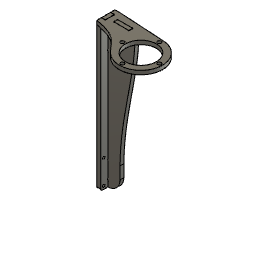
HoseSupport v3 (Autodesk Fusion 360 design; units mm, degrees)
Autodesk Fusion 360 part; units mm, degrees
sketch "Sketch1" plane through (0, 0, 0) normal (1, 0, 0) x (0, 0, -1)
  line L0 (0, 0) -> (10, 0) construction
  line L1 (10, 0) -> (50, 0) construction
  line L2 (10, 0) -> (10, 80) construction
  line L3 (50, 0) -> (50, 80) construction
  line L4 (0, 0) -> (0, -10) construction
  line L5 (0, 0) -> (0, 90) construction
  line L6 (0, 0) -> (60, 0) construction
  line L7 (60, 0) -> (60, 457.2) construction
  line L8 (0, -10) -> (60, -10)
  line L9 (60, -10) -> (60, 457.2)
  line L10 (60, 457.2) -> (0, 457.2)
  line L11 (0, 457.2) -> (0, -10)
  circle A0 centre (10, 80) radius 4
  circle A1 centre (50, 80) radius 4
  circle A2 centre (10, 0) radius 4
  circle A3 centre (50, 0) radius 4
  line L12 (30, -10) -> (30, 40) construction
  line L13 (36.35, 10) -> (23.65, 10)
  line L14 (23.65, 10) -> (23.65, 70)
  line L15 (23.65, 70) -> (36.35, 70)
  line L16 (36.35, 70) -> (36.35, 10)
  line L17 (36.35, 10) -> (23.65, 70) construction
  line L18 (23.65, 10) -> (36.35, 70) construction
  line L19 (30, 457.2) -> (30, 407.2) construction
  line L20 (36.35, 377.2) -> (23.65, 377.2)
  line L21 (23.65, 377.2) -> (23.65, 437.2)
  line L22 (23.65, 437.2) -> (36.35, 437.2)
  line L23 (36.35, 437.2) -> (36.35, 377.2)
  line L24 (36.35, 377.2) -> (23.65, 437.2) construction
  line L25 (23.65, 377.2) -> (36.35, 437.2) construction
  line L26 (0, 457.2) -> (15, 457.2) construction
  line L27 (60, 457.2) -> (45, 457.2) construction
  line L28 (45, 457.2) -> (45, 469.9) construction
  line L29 (15, 457.2) -> (45, 457.2)
  line L30 (45, 457.2) -> (45, 469.9)
  line L31 (45, 469.9) -> (15, 469.9)
  line L32 (15, 469.9) -> (15, 457.2)
  point P0 (30, 40)
  point P1 (30, 407.2)
  dimension "d1" = 10
  dimension "d2" = 40
  dimension "d3" = 80
  dimension "d4" = 80
  dimension "d5" = 10
  dimension "d6" = 90
  dimension "d8" = 60
  dimension "d9" = 457.2
  dimension "d10" = 8
  dimension "d11" = 8
  dimension "d12" = 8
  dimension "d13" = 8
  dimension "d14" = 50
  dimension "d15" = 12.7
  dimension "d16" = 60
  dimension "d17" = 50
  dimension "d18" = 12.7
  dimension "d19" = 60
  dimension "d20" = 15
  dimension "d21" = 15
  dimension "d22" = 12.7
  constraint coincident L0.start L4.start
  constraint horizontal L0
  constraint parallel L0 L1
  constraint perpendicular L1 L2
  constraint perpendicular L1 L3
  constraint perpendicular L0 L4
  constraint vertical L5
  constraint perpendicular L3 L6
  constraint perpendicular L6 L7
  constraint horizontal L8
  constraint vertical L9
  constraint horizontal L10
  constraint vertical L11
  constraint coincident L2.end A0.centre
  constraint coincident L3.end A1.centre
  constraint coincident L0.end L1.start
  constraint coincident L1.end L3.start
  constraint midpoint L8 L12.start
  constraint perpendicular L8 L12
  constraint horizontal L13
  constraint perpendicular L13 L14
  constraint parallel L13 L15
  constraint parallel L14 L16
  constraint coincident L17 P0
  constraint coincident L18 P0
  constraint coincident P0 L12.end
  constraint midpoint L10 L19.start
  constraint perpendicular L10 L19
  constraint horizontal L20
  constraint perpendicular L20 L21
  constraint parallel L20 L22
  constraint parallel L21 L23
  constraint coincident L24 P1
  constraint coincident L25 P1
  constraint coincident P1 L19.end
  constraint perpendicular L9 L26
  constraint perpendicular L9 L27
  constraint perpendicular L27 L28
  constraint horizontal L29
  constraint vertical L30
  constraint horizontal L31
  constraint vertical L32
  measures "d1" distance of L0.start L0.end
  measures "d2" distance of L0.end L1.end
  measures "d3" distance of L0.end L2.end
  measures "d4" distance of L1.end L3.end
  measures "d5" distance of L0.start L4.end
  measures "d6" distance of L0.start L5.end
  measures "d8" distance of L0.start L6.end
  measures "d9" distance of L6.end L7.end
  measures "d10" diameter of A0
  measures "d11" diameter of A1
  measures "d12" diameter of A2
  measures "d13" diameter of A3
  measures "d14" distance of L12.start P0
  measures "d15" distance of L14.end L15.end
  measures "d16" distance of L13.end L14.end
  measures "d17" distance of L19.start P1
  measures "d18" distance of L21.end L22.end
  measures "d19" distance of L20.end L21.end
  measures "d20" distance of L10.end L26.end
  measures "d21" distance of L7.end L27.end
  measures "d22" distance of L27.end L28.end
extrude "Extrude1" add sketch "Sketch1" along normal blind 12.7 makes body 1 in component "Component"
fillet "Fillet1" radius 6 2 edges at (6.35, -10, 0) (6.35, -10, -60) on bodies 1 in component "Component"
sketch "Sketch2" plane through (12.7, 0, 0) normal (1, 0, 0) x (0, 0, -1)
  arc A0 (54, -10) -> (60, -4) centre (54, -4) ccw
  line L0 (60, -4) -> (60, 457.2)
  line L1 (60, 457.2) -> (45, 457.2)
  line L2 (45, 457.2) -> (45, 469.9)
  line L3 (45, 469.9) -> (15, 469.9)
  line L4 (15, 469.9) -> (15, 457.2)
  line L5 (15, 457.2) -> (0, 457.2)
  line L6 (0, 457.2) -> (0, -4)
  arc A1 (0, -4) -> (6, -10) centre (6, -4) ccw
  line L7 (6, -10) -> (54, -10)
  circle A2 centre (50, 0) radius 4
  line L8 (23.65, 437.2) -> (36.35, 437.2)
  line L9 (36.35, 437.2) -> (36.35, 377.2)
  line L10 (36.35, 377.2) -> (23.65, 377.2)
  line L11 (23.65, 377.2) -> (23.65, 437.2)
  circle A3 centre (50, 80) radius 4
  circle A4 centre (10, 80) radius 4
  circle A5 centre (10, 0) radius 4
  line L12 (23.65, 70) -> (36.35, 70)
  line L13 (36.35, 70) -> (36.35, 10)
  line L14 (36.35, 10) -> (23.65, 10)
  line L15 (23.65, 10) -> (23.65, 70)
  line L16 (30, -10) -> (30, 223.6) construction
  line L17 (36.35, -10) -> (23.65, -10)
  line L18 (23.65, -10) -> (23.65, 457.2)
  line L19 (23.65, 457.2) -> (36.35, 457.2)
  line L20 (36.35, 457.2) -> (36.35, -10)
  line L21 (36.35, -10) -> (23.65, 457.2) construction
  line L22 (23.65, -10) -> (36.35, 457.2) construction
  point P0 (30, 223.6)
  dimension "d27" = 233.6
  dimension "d28" = 12.7
  constraint midpoint L7 L16.start
  constraint perpendicular L3 L16
  constraint horizontal L17
  constraint perpendicular L17 L18
  constraint parallel L17 L19
  constraint parallel L18 L20
  constraint coincident L21 P0
  constraint coincident L22 P0
  constraint coincident P0 L16.end
  measures "d27" distance of L16.start P0
  measures "d28" distance of L18.end L19.end
extrude "Extrude1'" add sketch "Sketch2" along normal blind 40 separate body contours L7 L14 L17 L18 L20 | L12 L13 L14 L15 L18 L20 | L10 L12 L18 L20 | L8 L9 L10 L11 L18 L20 | L8 L18 L19 L20 makes body 2 in component "Component'"
extrude "Extrude2" add sketch "Sketch2" against normal blind 12.7 contours L12 L13 L14 L15 L18 L20 | L8 L9 L10 L11 L18 L20 bodies 2 in component "Component'"
sketch "Sketch3" plane through (0, 0, -23.65) normal (0, 0, 1) x (1, 0, 0)
  line L0 (12.7, 10) -> (12.7, -10)
  line L1 (12.7, -10) -> (52.7, -10)
  line L2 (52.7, -10) -> (52.7, 457.2)
  line L3 (52.7, 457.2) -> (12.7, 457.2)
  line L4 (12.7, 457.2) -> (12.7, 437.2)
  line L5 (12.7, 437.2) -> (0, 437.2)
  line L6 (0, 437.2) -> (0, 377.2)
  line L7 (0, 377.2) -> (12.7, 377.2)
  line L8 (12.7, 377.2) -> (12.7, 70)
  line L9 (12.7, 70) -> (0, 70)
  line L10 (0, 70) -> (0, 10)
  line L11 (0, 10) -> (12.7, 10)
  line L12 (12.7, 457.2) -> (101.6, 457.2) construction
  line L13 (101.6, 457.2) -> (101.6, 384.9903)
  line L14 (101.6, 384.9903) -> (84.2206, 301.7516)
  line L15 (84.2206, 301.7516) -> (66.9638, 237.7998)
  line L16 (66.9638, 237.7998) -> (52.7, 146.4402)
  line L17 (52.7, 146.4402) -> (52.7, 70)
  spline S0 degree 5 poles (101.6, 457.2) (101.6, 384.9903) (84.2206, 301.7516) (66.9638, 237.7998) (52.7, 146.4402) (52.7, 70) knots 0 0 0 0 0 0 1 1 1 1 1 1
  line L18 (101.6, 457.2) -> (52.7, 457.2)
  dimension "d33" = 88.9
  constraint coincident L3.end L4.start
  constraint perpendicular L4 L12
  constraint coincident L2 L16.end
  constraint coincident L2 L17.end
  constraint coincident L2.end L3.start
  measures "d33" distance of L3.end L12.end
extrude "Extrude3" add sketch "Sketch3" against normal up to surface (12.7 mm away) contours L2 L15 L16 L17 S0 | L2 L15 L16 S0 L18 bodies 2 in component "Component'"
fillet "Fillet1'" radius 40 1 edges at (52.7, -10, -30) on bodies 2 in component "Component'"
sketch "Sketch4" plane through (0, 457.2, 0) normal (0, 1, 0) x (-1, 0, 0)
  line L0 (-12.7, -36.35) -> (-12.7, -23.65)
  line L1 (-12.7, -23.65) -> (-101.6, -23.65)
  line L2 (-101.6, -23.65) -> (-101.6, -36.35)
  line L3 (-101.6, -36.35) -> (-12.7, -36.35)
  line L4 (-57.15, -36.35) -> (-57.15, -30) construction
  line L5 (-82.15, -23.65) -> (-32.15, -23.65)
  line L6 (-32.15, -23.65) -> (-32.15, -36.35)
  line L7 (-32.15, -36.35) -> (-82.15, -36.35)
  line L8 (-82.15, -36.35) -> (-82.15, -23.65)
  line L9 (-82.15, -23.65) -> (-32.15, -36.35) construction
  line L10 (-32.15, -23.65) -> (-82.15, -36.35) construction
  point P0 (-57.15, -30)
  dimension "d38" = 6.35
  dimension "d39" = 50
  constraint midpoint L3 L4.start
  constraint perpendicular L1 L4
  constraint horizontal L5
  constraint perpendicular L5 L6
  constraint parallel L5 L7
  constraint parallel L6 L8
  constraint coincident L9 P0
  constraint coincident L10 P0
  constraint coincident P0 L4.end
  measures "d38" distance of L4.start P0
  measures "d39" distance of L6.end L7.end
extrude "Extrude4" add sketch "Sketch4" along normal blind 12.7 contours L1 L3 L5 L6 L7 L8 bodies 2 in component "Component'"
sketch "Sketch5" plane through (0, 457.2, 0) normal (0, 1, 0) x (-1, 0, 0)
  line L0 (0, -60) -> (0, -45)
  line L1 (0, -45) -> (-12.7, -45)
  line L2 (-12.7, -60) -> (0, -60)
  line L3 (-12.7, -45) -> (-12.7, -15)
  line L4 (-12.7, -15) -> (0, -15)
  line L5 (0, -15) -> (0, -45)
  line L6 (-12.7, -45) -> (-12.7, -36.35) construction
  line L7 (-12.7, -36.35) -> (-32.15, -36.35) construction
  line L8 (-32.15, -36.35) -> (-82.15, -36.35)
  line L9 (-82.15, -36.35) -> (-82.15, -23.65)
  line L10 (-82.15, -23.65) -> (-32.15, -23.65)
  line L11 (-32.15, -23.65) -> (-32.15, -36.35)
  line L12 (0, 0) -> (0, 20) construction
  line L13 (0, 20) -> (-165, 20) construction
  circle A0 centre (-165, 20) radius 50.8
  circle A1 centre (-165, 20) radius 70.8
  line L14 (0, 0) -> (-53.9716, 10)
  line L15 (-53.9716, 10) -> (-70, 20)
  line L16 (-70, 20) -> (-82.5, 32.0072)
  line L17 (-82.5, 32.0072) -> (-97.2493, 52.0068)
  line L18 (-97.2493, 52.0068) -> (-112.5505, 67.5572)
  spline S0 degree 5 poles (0, 0) (-53.9716, 10) (-70, 20) (-82.5, 32.0072) (-97.2493, 52.0068) (-112.5505, 67.5572) knots 0 0 0 0 0 0 1 1 1 1 1 1
  line L19 (0, 0) -> (0, -15)
  line L20 (-12.7, -60) -> (-169.211, -50.6747)
  dimension "d45" = 30
  dimension "d46" = 8.65
  dimension "d47" = 19.45
  dimension "d48" = 50
  dimension "d49" = 12.7
  dimension "d50" = 20
  dimension "d51" = 165
  dimension "d54" = 101.6
  dimension "d55" = 141.6
  constraint vertical L3
  constraint horizontal L4
  constraint vertical L5
  constraint coincident L0.end L1.start
  constraint coincident L1.end L3.start
  constraint perpendicular L3 L7
  constraint horizontal L8
  constraint vertical L9
  constraint horizontal L10
  constraint vertical L11
  constraint coincident L12.start L14.start
  constraint perpendicular L12 L13
  constraint coincident L13.end A0.centre
  constraint concentric A0 A1
  constraint coincident L13 L15.end
  constraint coincident A1 L18.end
  constraint coincident L2.start L20.start
  constraint coincident A1 L20.end
  constraint tangent A1 L20
  measures "d45" distance of L0.end L4.end
  measures "d46" distance of L1.end L6.end
  measures "d47" distance of L6.end L7.end
  measures "d48" distance of L7.end L8.end
  measures "d49" distance of L7.end L10.end
  measures "d50" distance of L12.start L12.end
  measures "d51" distance of L12.end L13.end
  measures "d54" diameter of A0
  measures "d55" diameter of A1
extrude "Extrude1''" add sketch "Sketch5" along normal blind 12.7 separate body contours L0 L1 L2 L3 L4 A1 L14 L15 L16 L17 S0 L19 L20 | A1 | L14 L15 L16 L17 S0 makes body 3 in component "Component''"
sketch "Sketch6" plane through (0, 469.9, 0) normal (0, 1, 0) x (-1, 0, 0)
  line L0 (-82.15, -23.65) -> (-32.15, -23.65)
  line L1 (-32.15, -23.65) -> (-32.15, -36.35)
  line L2 (-32.15, -36.35) -> (-82.15, -36.35)
  line L3 (-82.15, -36.35) -> (-82.15, -23.65)
  circle A0 centre (-165, 20) radius 50.8
  line L4 (0, -60) -> (0, -45)
  line L5 (0, -45) -> (-12.7, -45)
  line L6 (-12.7, -45) -> (-12.7, -15)
  line L7 (-12.7, -15) -> (0, -15)
  line L8 (0, -15) -> (0, 0)
  spline S0 degree 5 poles (0, 0) (-53.9716, 10) (-70, 20) (-82.5, 32.0072) (-97.2493, 52.0068) (-112.5505, 67.5572) knots 0 0 0 0 0 0 1 1 1 1 1 1
  arc A1 (-112.5505, 67.5572) -> (-169.211, -50.6747) centre (-165, 20) ccw
  line L9 (-169.211, -50.6747) -> (-12.7, -60)
  line L10 (-12.7, -60) -> (0, -60)
  line L11 (0, 0) -> (0, 20) construction
  line L12 (0, 20) -> (-165, 20) construction
  line L13 (-165, 20) -> (-165, -40.8) construction
  line L14 (-165, 20) -> (-225.8, 20) construction
  line L15 (-165, 20) -> (-225.8, 20) construction
  line L16 (-165, 20) -> (-165, 80.8) construction
  line L17 (-165, 20) -> (-104.2, 20) construction
  circle A2 centre (-165, -40.8) radius 6.0325
  circle A3 centre (-165, 80.8) radius 6.0325
  circle A4 centre (-225.8, 20) radius 6.0325
  line L18 (-165, 20) -> (-104.2, 20) construction
  circle A5 centre (-104.2, 20) radius 6.0325
  dimension "d58" = 20
  dimension "d59" = 165
  dimension "d60" = 60.8
  dimension "d61" = 360
  dimension "d62" = 60.8
  dimension "d63" = 90
  dimension "d64" = 60.8
  dimension "d65" = 12.065
  dimension "d66" = 12.065
  dimension "d67" = 12.065
  dimension "d70" = 12.065
  constraint coincident L8.end S0.start
  constraint parallel L8 L11
  constraint perpendicular L11 L12
  constraint perpendicular L12 L13
  constraint horizontal L15
  constraint coincident A0.centre A1.centre
  constraint horizontal L17
  constraint coincident L13.end A2.centre
  constraint coincident L16.end A3.centre
  constraint coincident L14.end L15.end
  constraint coincident L17.end L18.end
  measures "d58" distance of L8.end L11.end
  measures "d59" distance of L11.end A0.centre
  measures "d60" distance of A0.centre L13.end
  measures "d62" distance of A0.centre L14.end
  measures "d63" angle of L16 L17
  measures "d64" distance of A0.centre L16.end
  measures "d65" diameter of A2
  measures "d66" diameter of A3
  measures "d67" diameter of A4
  measures "d70" diameter of A5
extrude "Extrude2'" cut sketch "Sketch6" against normal blind 10.16 contours A2 | A3 | A4 bodies 3 in component "Component''"
extrude "Extrude3'" cut sketch "Sketch6" against normal blind 10.16 contours A5 bodies 3 in component "Component''"
ref_plane "WorkPlane1" through (0, 457.2, -15) normal (1, 0, 0) x (0, 1, 0)
sketch "Sketch7" plane through (0, 457.2, -15) normal (1, 0, 0) x (0, 1, 0)
  line L0 (12.7, 0) -> (0, 0) construction
  line L1 (0, 0) -> (0, 15) construction
  line L2 (0, 0) -> (2.2451, 2.2451) construction
  circle A0 centre (2.2451, 2.2451) radius 3.175
  dimension "d74" = 3.175
  constraint coincident L0.end L1.start
  constraint coincident L0.end A0
  measures "d74" distance of L0.end L2.end
sweep "Sweep1" cut kept parallel profiles "Sketch7" along 1 edges at (6.35, 457.2, -15) section 1 on bodies 1 bodies 1 in component "Component"
ref_plane "WorkPlane2" through (82.15, 457.2, -36.35) normal (0, 0, 1) x (1, 0, 0)
sketch "Sketch8" plane through (82.15, 457.2, -36.35) normal (0, 0, 1) x (1, 0, 0)
  line L0 (0, 0) -> (19.45, 0) construction
  line L1 (0, 0) -> (0, 12.7) construction
  line L2 (0, 0) -> (2.2451, 2.2451) construction
  circle A0 centre (2.2451, 2.2451) radius 3.175
  dimension "d82" = 3.175
  constraint coincident L0.start L1.start
  constraint coincident L0.start A0
  measures "d82" distance of L0.start L2.end
sweep "Sweep1'" cut kept parallel profiles "Sketch8" along 1 edges at (82.15, 457.2, -30) section 1 on bodies 2 bodies 2 in component "Component'"
ref_plane "WorkPlane3" through (32.15, 457.2, -23.65) normal (0, 0, -1) x (-1, 0, 0)
sketch "Sketch9" plane through (32.15, 457.2, -23.65) normal (0, 0, -1) x (-1, 0, 0)
  line L0 (19.45, 0) -> (0, 0) construction
  line L1 (0, 0) -> (0, 12.7) construction
  line L2 (0, 0) -> (2.2451, 2.2451) construction
  circle A0 centre (2.2451, 2.2451) radius 3.175
  dimension "d90" = 3.175
  constraint coincident L0.end L1.start
  constraint coincident L0.end A0
  measures "d90" distance of L0.end L2.end
sweep "Sweep2" cut kept parallel profiles "Sketch9" along 1 edges at (32.15, 457.2, -30) section 1 on bodies 2 bodies 2 in component "Component'"
ref_plane "WorkPlane4" through (0, 457.2, -45) normal (1, 0, 0) x (0, 1, 0)
sketch "Sketch10" plane through (0, 457.2, -45) normal (1, 0, 0) x (0, 1, 0)
  line L0 (0, -15) -> (0, 0) construction
  line L1 (0, 0) -> (12.7, 0) construction
  line L2 (0, 0) -> (2.2451, -2.2451) construction
  circle A0 centre (2.2451, -2.2451) radius 3.175
  dimension "d98" = 3.175
  constraint coincident L0.end L1.start
  constraint coincident L0.end A0
  measures "d98" distance of L0.end L2.end
sweep "Sweep2'" cut kept parallel profiles "Sketch10" along 1 edges at (6.35, 457.2, -45) section 1 on bodies 1 bodies 1 in component "Component"
ref_plane "WorkPlane5" through (12.7, 437.2, -36.35) normal (0, 0, 1) x (1, 0, 0)
sketch "Sketch11" plane through (12.7, 437.2, -36.35) normal (0, 0, 1) x (1, 0, 0)
  line L0 (0, 0) -> (0, 20) construction
  line L1 (0, 0) -> (-12.7, 0) construction
  line L2 (0, 0) -> (-2.2451, 2.2451) construction
  circle A0 centre (-2.2451, 2.2451) radius 3.175
  dimension "d106" = 3.175
  constraint coincident L0.start L1.start
  constraint coincident L0.start A0
  measures "d106" distance of L0.start L2.end
sweep "Sweep3" cut kept parallel profiles "Sketch11" along 1 edges at (12.7, 437.2, -30) section 1 on bodies 2 bodies 2 in component "Component'"
ref_plane "WorkPlane6" through (12.7, 377.2, -23.65) normal (0, 0, -1) x (-1, 0, 0)
sketch "Sketch12" plane through (12.7, 377.2, -23.65) normal (0, 0, -1) x (-1, 0, 0)
  line L0 (0, -307.2) -> (0, 0) construction
  line L1 (0, 0) -> (12.7, 0) construction
  line L2 (0, 0) -> (2.2451, -2.2451) construction
  circle A0 centre (2.2451, -2.2451) radius 3.175
  dimension "d114" = 3.175
  constraint coincident L0.end L1.start
  constraint coincident L0.end A0
  measures "d114" distance of L0.end L2.end
sweep "Sweep4" cut kept parallel profiles "Sketch12" along 1 edges at (12.7, 377.2, -30) section 1 on bodies 2 bodies 2 in component "Component'"
ref_plane "WorkPlane7" through (12.7, 10, -23.65) normal (0, 0, -1) x (-1, 0, 0)
sketch "Sketch13" plane through (12.7, 10, -23.65) normal (0, 0, -1) x (-1, 0, 0)
  line L0 (0, 0) -> (0, -20) construction
  line L1 (0, 0) -> (12.7, 0) construction
  line L2 (0, 0) -> (2.2451, -2.2451) construction
  circle A0 centre (2.2451, -2.2451) radius 3.175
  dimension "d122" = 3.175
  constraint coincident L0.start L1.start
  constraint coincident L0.start A0
  measures "d122" distance of L0.start L2.end
sweep "Sweep5" cut kept parallel profiles "Sketch13" along 1 edges at (12.7, 10, -30) section 1 on bodies 2 bodies 2 in component "Component'"
ref_plane "WorkPlane8" through (12.7, 70, -36.35) normal (0, 0, 1) x (1, 0, 0)
sketch "Sketch14" plane through (12.7, 70, -36.35) normal (0, 0, 1) x (1, 0, 0)
  line L0 (0, 302.7099) -> (0, 0) construction
  line L1 (0, 0) -> (-12.7, 0) construction
  line L2 (0, 0) -> (-2.2451, 2.2451) construction
  circle A0 centre (-2.2451, 2.2451) radius 3.175
  dimension "d130" = 3.175
  constraint coincident L0.end L1.start
  constraint coincident L0.end A0
  measures "d130" distance of L0.end L2.end
sweep "Sweep6" cut kept parallel profiles "Sketch14" along 1 edges at (12.7, 70, -30) section 1 on bodies 2 bodies 2 in component "Component'"
ref_plane "WorkPlane9" through (0, 377.2, -23.65) normal (1, 0, 0) x (0, 1, 0)
sketch "Sketch15" plane through (0, 377.2, -23.65) normal (1, 0, 0) x (0, 1, 0)
  line L0 (0, -12.7) -> (0, 0) construction
  line L1 (0, 0) -> (60, 0) construction
  line L2 (0, 0) -> (2.2451, -2.2451) construction
  circle A0 centre (2.2451, -2.2451) radius 3.175
  dimension "d138" = 3.175
  constraint coincident L0.end L1.start
  constraint coincident L0.end A0
  measures "d138" distance of L0.end L2.end
sweep "Sweep3'" cut kept parallel profiles "Sketch15" along 1 edges at (6.35, 377.2, -23.65) section 1 on bodies 1 bodies 1 in component "Component"
ref_plane "WorkPlane10" through (0, 437.2, -23.65) normal (1, 0, 0) x (0, 1, 0)
sketch "Sketch16" plane through (0, 437.2, -23.65) normal (1, 0, 0) x (0, 1, 0)
  line L0 (0, 0) -> (0, -12.7) construction
  line L1 (-55.5099, 0) -> (0, 0) construction
  line L2 (0, 0) -> (-2.2451, -2.2451) construction
  circle A0 centre (-2.2451, -2.2451) radius 3.175
  dimension "d146" = 3.175
  constraint coincident L0.start L1.end
  constraint coincident L0.start A0
  measures "d146" distance of L0.start L2.end
sweep "Sweep4'" cut kept parallel profiles "Sketch16" along 1 edges at (6.35, 437.2, -23.65) section 1 on bodies 1 bodies 1 in component "Component"
ref_plane "WorkPlane11" through (0, 437.2, -36.35) normal (1, 0, 0) x (0, 1, 0)
sketch "Sketch17" plane through (0, 437.2, -36.35) normal (1, 0, 0) x (0, 1, 0)
  line L0 (0, 8.2099) -> (0, 0) construction
  line L1 (0, 0) -> (-60, 0) construction
  line L2 (0, 0) -> (-2.2451, 2.2451) construction
  circle A0 centre (-2.2451, 2.2451) radius 3.175
  dimension "d154" = 3.175
  constraint coincident L0.end L1.start
  constraint coincident L0.end A0
  measures "d154" distance of L0.end L2.end
sweep "Sweep5'" cut kept parallel profiles "Sketch17" along 1 edges at (6.35, 437.2, -36.35) section 1 on bodies 1 bodies 1 in component "Component"
ref_plane "WorkPlane12" through (0, 377.2, -36.35) normal (1, 0, 0) x (0, 1, 0)
sketch "Sketch18" plane through (0, 377.2, -36.35) normal (1, 0, 0) x (0, 1, 0)
  line L0 (55.5099, 0) -> (0, 0) construction
  line L1 (0, 0) -> (0, 8.2099) construction
  line L2 (0, 0) -> (2.2451, 2.2451) construction
  circle A0 centre (2.2451, 2.2451) radius 3.175
  dimension "d162" = 3.175
  constraint coincident L0.end L1.start
  constraint coincident L0.end A0
  measures "d162" distance of L0.end L2.end
sweep "Sweep6'" cut kept parallel profiles "Sketch18" along 1 edges at (6.35, 377.2, -36.35) section 1 on bodies 1 bodies 1 in component "Component"
ref_plane "WorkPlane13" through (0, 10, -36.35) normal (1, 0, 0) x (0, 1, 0)
sketch "Sketch19" plane through (0, 10, -36.35) normal (1, 0, 0) x (0, 1, 0)
  line L0 (60, 0) -> (0, 0) construction
  line L1 (0, 0) -> (0, 12.7) construction
  line L2 (0, 0) -> (2.2451, 2.2451) construction
  circle A0 centre (2.2451, 2.2451) radius 3.175
  dimension "d170" = 3.175
  constraint coincident L0.end L1.start
  constraint coincident L0.end A0
  measures "d170" distance of L0.end L2.end
sweep "Sweep7" cut kept parallel profiles "Sketch19" along 1 edges at (6.35, 10, -36.35) section 1 on bodies 1 bodies 1 in component "Component"
ref_plane "WorkPlane14" through (0, 10, -23.65) normal (1, 0, 0) x (0, 1, 0)
sketch "Sketch20" plane through (0, 10, -23.65) normal (1, 0, 0) x (0, 1, 0)
  line L0 (0, -8.2099) -> (0, 0) construction
  line L1 (0, 0) -> (60, 0) construction
  line L2 (0, 0) -> (2.2451, -2.2451) construction
  circle A0 centre (2.2451, -2.2451) radius 3.175
  dimension "d178" = 3.175
  constraint coincident L0.end L1.start
  constraint coincident L0.end A0
  measures "d178" distance of L0.end L2.end
sweep "Sweep8" cut kept parallel profiles "Sketch20" along 1 edges at (6.35, 10, -23.65) section 1 on bodies 1 bodies 1 in component "Component"
ref_plane "WorkPlane15" through (0, 70, -23.65) normal (1, 0, 0) x (0, 1, 0)
sketch "Sketch21" plane through (0, 70, -23.65) normal (1, 0, 0) x (0, 1, 0)
  line L0 (0, 0) -> (0, -12.7) construction
  line L1 (-55.5099, 0) -> (0, 0) construction
  line L2 (0, 0) -> (-2.2451, -2.2451) construction
  circle A0 centre (-2.2451, -2.2451) radius 3.175
  dimension "d186" = 3.175
  constraint coincident L0.start L1.end
  constraint coincident L0.start A0
  measures "d186" distance of L0.start L2.end
sweep "Sweep9" cut kept parallel profiles "Sketch21" along 1 edges at (6.35, 70, -23.65) section 1 on bodies 1 bodies 1 in component "Component"
ref_plane "WorkPlane16" through (0, 70, -36.35) normal (1, 0, 0) x (0, 1, 0)
sketch "Sketch22" plane through (0, 70, -36.35) normal (1, 0, 0) x (0, 1, 0)
  line L0 (0, 8.2099) -> (0, 0) construction
  line L1 (0, 0) -> (-55.5099, 0) construction
  line L2 (0, 0) -> (-2.2451, 2.2451) construction
  circle A0 centre (-2.2451, 2.2451) radius 3.175
  dimension "d194" = 3.175
  constraint coincident L0.end L1.start
  constraint coincident L0.end A0
  measures "d194" distance of L0.end L2.end
sweep "Sweep10" cut kept parallel profiles "Sketch22" along 1 edges at (6.35, 70, -36.35) section 1 on bodies 1 bodies 1 in component "Component"
ref_plane "WorkPlane17" through (12.7, 457.2, -45) normal (0, 1, 0) x (-1, 0, 0)
sketch "Sketch23" plane through (12.7, 457.2, -45) normal (0, 1, 0) x (-1, 0, 0)
  line L0 (12.7, 0) -> (0, 0) construction
  line L1 (0, 0) -> (0, 30) construction
  line L2 (0, 0) -> (2.2451, 2.2451) construction
  circle A0 centre (2.2451, 2.2451) radius 3.175
  dimension "d202" = 3.175
  constraint coincident L0.end L1.start
  constraint coincident L0.end A0
  measures "d202" distance of L0.end L2.end
sweep "Sweep1''" cut kept parallel profiles "Sketch23" along 1 edges at (12.7, 463.55, -45) section 1 on bodies 3 bodies 3 in component "Component''"
ref_plane "WorkPlane18" through (12.7, 457.2, -15) normal (0, 1, 0) x (-1, 0, 0)
sketch "Sketch24" plane through (12.7, 457.2, -15) normal (0, 1, 0) x (-1, 0, 0)
  line L0 (0, -25.5099) -> (0, 0) construction
  line L1 (0, 0) -> (12.7, 0) construction
  line L2 (0, 0) -> (2.2451, -2.2451) construction
  circle A0 centre (2.2451, -2.2451) radius 3.175
  dimension "d210" = 3.175
  constraint coincident L0.end L1.start
  constraint coincident L0.end A0
  measures "d210" distance of L0.end L2.end
sweep "Sweep2''" cut kept parallel profiles "Sketch24" along 1 edges at (12.7, 463.55, -15) section 1 on bodies 3 bodies 3 in component "Component''"
ref_plane "WorkPlane19" through (82.15, 457.2, -23.65) normal (0, 1, 0) x (-1, 0, 0)
sketch "Sketch25" plane through (82.15, 457.2, -23.65) normal (0, 1, 0) x (-1, 0, 0)
  line L0 (0, 0) -> (50, 0) construction
  line L1 (0, -12.7) -> (0, 0) construction
  line L2 (0, 0) -> (2.2451, -2.2451) construction
  circle A0 centre (2.2451, -2.2451) radius 3.175
  dimension "d218" = 3.175
  constraint coincident L0.start L1.end
  constraint coincident L0.start A0
  measures "d218" distance of L0.start L2.end
sweep "Sweep3''" cut kept parallel profiles "Sketch25" along 1 edges at (82.15, 463.55, -23.65) section 1 on bodies 3 bodies 3 in component "Component''"
ref_plane "WorkPlane20" through (82.15, 457.2, -36.35) normal (0, 1, 0) x (-1, 0, 0)
sketch "Sketch26" plane through (82.15, 457.2, -36.35) normal (0, 1, 0) x (-1, 0, 0)
  line L0 (50, 0) -> (0, 0) construction
  line L1 (0, 0) -> (0, 8.2099) construction
  line L2 (0, 0) -> (2.2451, 2.2451) construction
  circle A0 centre (2.2451, 2.2451) radius 3.175
  dimension "d226" = 3.175
  constraint coincident L0.end L1.start
  constraint coincident L0.end A0
  measures "d226" distance of L0.end L2.end
sweep "Sweep4''" cut kept parallel profiles "Sketch26" along 1 edges at (82.15, 463.55, -36.35) section 1 on bodies 3 bodies 3 in component "Component''"
ref_plane "WorkPlane21" through (32.15, 457.2, -36.35) normal (0, 1, 0) x (-1, 0, 0)
sketch "Sketch27" plane through (32.15, 457.2, -36.35) normal (0, 1, 0) x (-1, 0, 0)
  line L0 (0, 12.7) -> (0, 0) construction
  line L1 (0, 0) -> (-45.5099, 0) construction
  line L2 (0, 0) -> (-2.2451, 2.2451) construction
  circle A0 centre (-2.2451, 2.2451) radius 3.175
  dimension "d234" = 3.175
  constraint coincident L0.end L1.start
  constraint coincident L0.end A0
  measures "d234" distance of L0.end L2.end
sweep "Sweep5''" cut kept parallel profiles "Sketch27" along 1 edges at (32.15, 463.55, -36.35) section 1 on bodies 3 bodies 3 in component "Component''"
ref_plane "WorkPlane22" through (32.15, 457.2, -23.65) normal (0, 1, 0) x (-1, 0, 0)
sketch "Sketch28" plane through (32.15, 457.2, -23.65) normal (0, 1, 0) x (-1, 0, 0)
  line L0 (-45.5099, 0) -> (0, 0) construction
  line L1 (0, 0) -> (0, -8.2099) construction
  line L2 (0, 0) -> (-2.2451, -2.2451) construction
  circle A0 centre (-2.2451, -2.2451) radius 3.175
  dimension "d242" = 3.175
  constraint coincident L0.end L1.start
  constraint coincident L0.end A0
  measures "d242" distance of L0.end L2.end
sweep "Sweep6''" cut kept parallel profiles "Sketch28" along 1 edges at (32.15, 463.55, -23.65) section 1 on bodies 3 bodies 3 in component "Component''"
component "Component" placed x (1, 0, 0) y (0, 1, 0) z (0, 0, 1) at (0, 0, 0)
component "Component'" placed x (1, 0, 0) y (0, 1, 0) z (0, 0, 1) at (0, 0, 0)
component "Component''" placed x (1, 0, 0) y (0, 1, 0) z (0, 0, 1) at (0, 0, 0)
equation "d27 = ( 479.900 mm - 0.5 in ) / 2"
equation "d38 = ( 12.700 / 2 ) * 1 mm"
equation "d46 = 15 mm - 0.25 in"
equation "hosediam = 4 in"
equation "d54 = hosediam"
equation "d55 = hosediam + 40 mm"
equation "d60 = hosediam / 2 + 10 mm"
equation "d62 = hosediam / 2 + 10 mm"
equation "d64 = hosediam / 2 + 10 mm"
equation "d74 = 0.25 in / 2"
equation "d82 = 0.25 in / 2"
equation "d90 = 0.25 in / 2"
equation "d98 = 0.25 in / 2"
equation "d106 = 0.25 in / 2"
equation "d114 = 0.25 in / 2"
equation "d122 = 0.25 in / 2"
equation "d130 = 0.25 in / 2"
equation "d138 = 0.25 in / 2"
equation "d146 = 0.25 in / 2"
equation "d154 = 0.25 in / 2"
equation "d162 = 0.25 in / 2"
equation "d170 = 0.25 in / 2"
equation "d178 = 0.25 in / 2"
equation "d186 = 0.25 in / 2"
equation "d194 = 0.25 in / 2"
equation "d202 = 0.25 in / 2"
equation "d210 = 0.25 in / 2"
equation "d218 = 0.25 in / 2"
equation "d226 = 0.25 in / 2"
equation "d234 = 0.25 in / 2"
equation "d242 = 0.25 in / 2"
